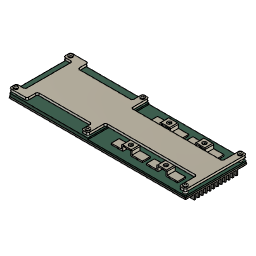
BMS (Autodesk Fusion 360 design; units mm, degrees)
Autodesk Fusion 360 part; units mm, degrees
note: some values were not read from the file. Set by a fixed rule: which sketch regions a step uses.
sketch "Sketch1" plane through (0, 0, 0) normal (0, 0, 1) x (1, 0, 0)
  line L0 (0, 0) -> (220, 0)
  line L1 (220, 0) -> (220, 76.5)
  line L2 (220, 76.5) -> (0, 76.5)
  line L3 (0, 76.5) -> (0, 0)
  line L4 (0, 38.25) -> (0, 65.25)
  line L5 (0, 38.25) -> (0, 11.25)
  line L6 (0, 11.25) -> (220, 11.25)
  line L7 (0, 65.25) -> (220, 65.25)
  line L8 (220, 0) -> (212, 0)
  line L9 (212, 0) -> (212, 76.5)
  line L10 (212, 38.25) -> (212, 54.25)
  line L11 (212, 38.25) -> (212, 22.25)
  line L12 (212, 22.25) -> (98, 22.25)
  line L13 (98, 22.25) -> (98, 54.25)
  line L14 (98, 54.25) -> (212, 54.25)
  line L15 (98, 54.25) -> (98, 76.5)
  line L16 (98, 22.25) -> (98, 0)
  line L17 (98, 0) -> (90, 0)
  line L18 (98, 76.5) -> (90, 76.5)
  line L19 (0, 0) -> (1.6578, 0)
  line L20 (0, 0) -> (22, 0)
  line L21 (0, 76.5) -> (22, 76.5)
  line L22 (22, 76.5) -> (22, 65.5)
  line L23 (24, 63.5) -> (88, 63.5)
  line L24 (90, 65.5) -> (90, 76.5)
  line L25 (22, 0) -> (22, 11)
  line L26 (24, 13) -> (88, 13)
  line L27 (90, 11) -> (90, 0)
  line L28 (0, 38.25) -> (0, 67.75)
  line L29 (0, 38.25) -> (0, 8.75)
  line L30 (0, 8.75) -> (9, 8.75)
  line L31 (11, 10.75) -> (11, 65.75)
  line L32 (9, 67.75) -> (0, 67.75)
  arc A0 (11, 65.75) -> (9, 67.75) centre (9, 65.75) ccw
  arc A1 (9, 8.75) -> (11, 10.75) centre (9, 10.75) ccw
  arc A2 (24, 13) -> (22, 11) centre (24, 11) ccw
  arc A3 (90, 11) -> (88, 13) centre (88, 11) ccw
  arc A4 (88, 63.5) -> (90, 65.5) centre (88, 65.5) ccw
  arc A5 (22, 65.5) -> (24, 63.5) centre (24, 65.5) ccw
  line L33 (94, 0) -> (94, 4)
  line L34 (0, 0) -> (4, 0)
  line L35 (4, 0) -> (4, 4)
  line L36 (4, 4) -> (0, 4)
  line L37 (0, 4) -> (0, 0)
  line L38 (216, 0) -> (216, 4)
  circle A6 centre (94, 4) radius 2.5
  circle A7 centre (4, 4) radius 2.5
  circle A8 centre (216, 4) radius 2.5
  line L39 (212, 76.5) -> (220, 76.5)
  line L40 (216, 76.5) -> (216, 72.5)
  circle A9 centre (216, 72.5) radius 2.5
  line L41 (94, 76.5) -> (94, 72.5)
  circle A10 centre (94, 72.5) radius 2.5
  line L42 (0, 76.5) -> (4, 76.5)
  line L43 (4, 76.5) -> (4, 72.5)
  line L44 (4, 72.5) -> (0, 72.5)
  line L45 (0, 72.5) -> (0, 76.5)
  circle A11 centre (4, 72.5) radius 2.5
  point P0 (22, 63.5)
  point P1 (22, 13)
  point P2 (11, 8.75)
  dimension "d1" = 220
  dimension "d2" = 76.5
  dimension "d3" = 27
  dimension "d4" = 27
  dimension "d5" = 8
  dimension "d6" = 16
  dimension "d7" = 16
  dimension "d8" = 114
  dimension "d9" = 8
  dimension "d10" = 8
  dimension "d11" = 22
  dimension "d12" = 22
  dimension "d13" = 13
  dimension "d14" = 13
  dimension "d15" = 29.5
  dimension "d16" = 29.5
  dimension "d17" = 11
  dimension "d18" = 2
  dimension "d19" = 4
  dimension "d20" = 4
  dimension "d21" = 4
  dimension "d22" = 4
  dimension "d23" = 5
  dimension "d24" = 5
  dimension "d25" = 5
  dimension "d26" = 4
  dimension "d27" = 5
  dimension "d28" = 4
  dimension "d29" = 5
  dimension "d30" = 4
  dimension "d31" = 4
  dimension "d32" = 5
  constraint horizontal L0
  constraint vertical L1
  constraint horizontal L2
  constraint vertical L3
  constraint coincident L0.start L3.end
  constraint midpoint L3 L4.start
  constraint parallel L3 L4
  constraint parallel L3 L5
  constraint coincident L1 L6.end
  constraint perpendicular L1 L6
  constraint coincident L1 L7.end
  constraint perpendicular L1 L7
  constraint perpendicular L1 L8
  constraint coincident L2 L9.end
  constraint perpendicular L2 L9
  constraint midpoint L9 L10.start
  constraint perpendicular L7 L10
  constraint parallel L9 L11
  constraint perpendicular L11 L12
  constraint perpendicular L6 L13
  constraint perpendicular L9 L14
  constraint coincident L2 L15.end
  constraint perpendicular L2 L15
  constraint coincident L0 L16.end
  constraint perpendicular L0 L16
  constraint coincident L0 L17.end
  constraint coincident L2 L18.end
  constraint coincident L0 L19.end
  constraint perpendicular L3 L20
  constraint perpendicular L3 L21
  constraint perpendicular L21 L22
  constraint perpendicular L22 L23
  constraint perpendicular L18 L24
  constraint perpendicular L6 L25
  constraint perpendicular L25 L26
  constraint perpendicular L17 L27
  constraint perpendicular L3 L30
  constraint perpendicular L7 L31
  constraint perpendicular L28 L32
  constraint tangent L31 A0
  constraint tangent L32 A0
  constraint coincident P2 L30
  constraint coincident P2 L31
  constraint tangent L30 A1
  constraint tangent L31 A1
  constraint equal A0 A1
  constraint coincident P1 L25
  constraint coincident P1 L26
  constraint tangent L25 A2
  constraint tangent L26 A2
  constraint equal A0 A2
  constraint tangent L26 A3
  constraint tangent L27 A3
  constraint equal A0 A3
  constraint tangent L23 A4
  constraint tangent L24 A4
  constraint equal A0 A4
  constraint coincident P0 L22
  constraint coincident P0 L23
  constraint tangent L22 A5
  constraint tangent L23 A5
  constraint equal A0 A5
  constraint midpoint L17 L33.start
  constraint perpendicular L0 L33
  constraint horizontal L34
  constraint vertical L35
  constraint horizontal L36
  constraint vertical L37
  constraint midpoint L8 L38.start
  constraint perpendicular L8 L38
  constraint coincident L33.end A6.centre
  constraint coincident L35.end L36.start
  constraint coincident L38.end A8.centre
  constraint midpoint L39 L40.start
  constraint perpendicular L39 L40
  constraint coincident L40.end A9.centre
  constraint midpoint L18 L41.start
  constraint perpendicular L18 L41
  constraint coincident L41.end A10.centre
  constraint horizontal L42
  constraint vertical L43
  constraint horizontal L44
  constraint vertical L45
  constraint coincident L43.end L44.start
  measures "d1" distance of L0.start L0.end
  measures "d2" distance of L0.start L2.end
  measures "d3" distance of L4.start L4.end
  measures "d4" distance of L4.start L5.end
  measures "d5" distance of L0.end L8.end
  measures "d6" distance of L10.start L10.end
  measures "d7" distance of L10.start L11.end
  measures "d8" distance of L11.end L12.end
  measures "d9" distance of L16.end L17.end
  measures "d10" distance of L15.end L18.end
  measures "d11" distance of L0.start L20.end
  measures "d12" distance of L2.end L21.end
  measures "d13" distance of L21.end P0
  measures "d14" distance of L20.end P1
  measures "d15" distance of L4.start L28.end
  measures "d16" distance of L4.start L29.end
  measures "d17" distance of L29.end P2
  measures "d18" radius of A0
  measures "d19" distance of L33.start L33.end
  measures "d20" distance of L0.start L34.end
  measures "d21" distance of L0.start L36.end
  measures "d22" distance of L38.start L38.end
  measures "d23" diameter of A6
  measures "d24" diameter of A7
  measures "d25" diameter of A8
  measures "d26" distance of L40.start L40.end
  measures "d27" diameter of A9
  measures "d28" distance of L41.start L41.end
  measures "d29" diameter of A10
  measures "d30" distance of L2.end L42.end
  measures "d31" distance of L2.end L44.end
  measures "d32" diameter of A11
extrude "Extrude1" add sketch "Sketch1" against normal blind 2 contours L0 L3 L19 L20 L34 L35 L36 L37 A7 | L0 L3 L6 L20 L25 L30 L31 A1 A2 L35 L36 A7 | L3 L6 L29 L30 L31 A1 | L35 L36 A7 | L35 L36 A7 | L0 L6 L25 L27 A2 A3 | L3 L4 L5 L6 L7 L28 L29 L31 | L0 L6 L16 L17 L27 A3 | L6 L7 L13 L15 L16 L23 L26 L31 A2 A3 A4 A5 | L6 L26 A2 A3 | L3 L7 L28 L31 L32 A0 | L2 L3 L7 L21 L22 L31 L32 A0 A5 L43 L44 A11 | L0 L6 L9 L16 | L2 L7 L22 L24 A4 A5 | L7 L23 A4 A5 | L0 L1 L6 L8 L9 | L6 L9 L12 L16 | L2 L3 L21 L42 L43 L44 L45 A11 | L2 L7 L15 L18 L24 A4 | L1 L6 L7 L9 L10 L11 | L9 L10 L11 L12 L13 L14 | L43 L44 A11 | L43 L44 A11 | L2 L7 L9 L15 | L7 L9 L14 L15 | L1 L2 L7 L9 L39 | A6 | A8 | A9 | A10 makes body 1
extrude "Extrude2" add sketch "Sketch1" along normal blind 4 and the other way blind -7 separate body contours L0 L3 L19 L20 L34 L35 L36 L37 A7 | L0 L3 L6 L20 L25 L30 L31 A1 A2 L35 L36 A7 | L35 L36 A7 | L35 L36 A7 | L0 L6 L16 L17 L27 A3 | L6 L7 L13 L15 L16 L23 L26 L31 A2 A3 A4 A5 | L2 L3 L7 L21 L22 L31 L32 A0 A5 L43 L44 A11 | L0 L1 L6 L8 L9 | L2 L3 L21 L42 L43 L44 L45 A11 | L2 L7 L15 L18 L24 A4 | L1 L6 L7 L9 L10 L11 | L9 L10 L11 L12 L13 L14 | L43 L44 A11 | L43 L44 A11 | L1 L2 L7 L9 L39 | A6 | A8 | A9 | A10 makes body 2
fillet "Fillet1" radius 2 18 edges at (98, 22.25, 5.5) (98, 54.25, 5.5) (212, 54.25, 5.5) (212, 22.25, 5.5) (212, 76.5, 5.5) (220, 76.5, 5.5) (212, 0, 5.5) (220, 0, 5.5) (98, 76.5, 5.5) (90, 76.5, 5.5) (98, 0, 5.5) (90, 0, 5.5) (22, 76.5, 5.5) (0, 76.5, 5.5) (0, 67.75, 5.5) (0, 8.75, 5.5) (0, 0, 5.5) (22, 0, 5.5) on bodies 2
extrude "Extrude3" add sketch "Sketch1" along normal blind 7 and the other way blind -9 contours L35 L36 A7 | L35 L36 A7 | L43 L44 A11 | L43 L44 A11 | A6 | A8 | A9 | A10 bodies 2
fillet "Fillet2" radius 1 6 edges at (1.6692, 71.596, 9) (1.6692, 3.096, 9) (91.6692, 3.096, 9) (91.6692, 71.596, 9) (213.6692, 3.096, 9) (213.6692, 71.596, 9) on bodies 2
extrude "Extrude4" add sketch "Sketch1" along normal blind 1.6 contours L0 L3 L19 L20 L34 L35 L36 L37 A7 | L0 L3 L6 L20 L25 L30 L31 A1 A2 L35 L36 A7 | L3 L6 L29 L30 L31 A1 | L35 L36 A7 | L35 L36 A7 | L0 L6 L25 L27 A2 A3 | L3 L4 L5 L6 L7 L28 L29 L31 | L0 L6 L16 L17 L27 A3 | L6 L7 L13 L15 L16 L23 L26 L31 A2 A3 A4 A5 | L6 L26 A2 A3 | L3 L7 L28 L31 L32 A0 | L2 L3 L7 L21 L22 L31 L32 A0 A5 L43 L44 A11 | L2 L7 L22 L24 A4 A5 | L7 L23 A4 A5 | L2 L3 L21 L42 L43 L44 L45 A11 | L2 L7 L15 L18 L24 A4 | L43 L44 A11 | L43 L44 A11 | A6 | A10 bodies 1
extrude "Extrude5" add sketch "Sketch1" along normal blind 4 contours L35 L36 A7 | L35 L36 A7 | L43 L44 A11 | L43 L44 A11 | A6 | A8 | A9 | A10 bodies 2
fillet "Fillet3" radius 1 4 edges at (220, 76.5, -1) (220, 0, -1) (0, 0, -1) (0, 76.5, -1) on bodies 1
extrude "Extrude6" add sketch "Sketch1" along normal blind -2 and the other way blind 4 separate body contours L0 L3 L19 L20 L34 L35 L36 L37 A7 | L0 L3 L6 L20 L25 L30 L31 A1 A2 L35 L36 A7 | L3 L6 L29 L30 L31 A1 | L35 L36 A7 | L35 L36 A7 | L0 L6 L25 L27 A2 A3 | L3 L4 L5 L6 L7 L28 L29 L31 | L0 L6 L16 L17 L27 A3 | L6 L7 L13 L15 L16 L23 L26 L31 A2 A3 A4 A5 | L6 L26 A2 A3 | L3 L7 L28 L31 L32 A0 | L2 L3 L7 L21 L22 L31 L32 A0 A5 L43 L44 A11 | L0 L6 L9 L16 | L2 L7 L22 L24 A4 A5 | L7 L23 A4 A5 | L0 L1 L6 L8 L9 | L6 L9 L12 L16 | L2 L3 L21 L42 L43 L44 L45 A11 | L2 L7 L15 L18 L24 A4 | L1 L6 L7 L9 L10 L11 | L9 L10 L11 L12 L13 L14 | L43 L44 A11 | L43 L44 A11 | L2 L7 L9 L15 | L7 L9 L14 L15 | L1 L2 L7 L9 L39 | A6 | A8 | A9 | A10 makes body 3
sketch "Sketch2" plane through (0, 0, -4) normal (0, 0, -1) x (1, 0, 0)
  line L0 (0, 0) -> (0, -76.5)
  line L1 (0, -76.5) -> (220, -76.5)
  line L2 (220, -76.5) -> (220, 0)
  line L3 (220, 0) -> (0, 0)
  line L4 (0, -38.25) -> (0, -11.25)
  line L5 (0, -38.25) -> (0, -65.25)
  line L6 (0, -65.25) -> (220, -65.25)
  line L7 (0, -11.25) -> (220, -11.25)
  line L8 (0, -65.25) -> (0, -63.5)
  line L9 (0, -63.5) -> (0, -60.5)
  line L10 (0, -60.5) -> (0, -58.75)
  line L11 (0, -58.75) -> (0, -55.75)
  line L12 (0, -55.75) -> (0, -54)
  line L13 (0, -54) -> (0, -51)
  line L14 (0, -51) -> (0, -49.25)
  line L15 (0, -49.25) -> (0, -46.25)
  line L16 (0, -46.25) -> (0, -44.5)
  line L17 (0, -44.5) -> (0, -41.5)
  line L18 (0, -41.5) -> (0, -39.75)
  line L19 (0, -39.75) -> (0, -38.25)
  line L20 (0, -11.25) -> (0, -13)
  line L21 (0, -13) -> (0, -16)
  line L22 (0, -16) -> (0, -17.75)
  line L23 (0, -17.75) -> (0, -20.75)
  line L24 (0, -20.75) -> (0, -22.5)
  line L25 (0, -22.5) -> (0, -25.5)
  line L26 (0, -25.5) -> (0, -27.25)
  line L27 (0, -27.25) -> (0, -30.25)
  line L28 (0, -30.25) -> (0, -32)
  line L29 (0, -32) -> (0, -35)
  line L30 (0, -35) -> (0, -36.75)
  line L31 (0, -63.5) -> (220, -63.5)
  line L32 (0, -60.5) -> (220, -60.5)
  line L33 (0, -58.75) -> (220, -58.75)
  line L34 (0, -55.75) -> (220, -55.75)
  line L35 (0, -54) -> (220, -54)
  line L36 (0, -51) -> (220, -51)
  line L37 (0, -49.25) -> (220, -49.25)
  line L38 (0, -46.25) -> (220, -46.25)
  line L39 (0, -44.5) -> (220, -44.5)
  line L40 (0, -41.5) -> (220, -41.5)
  line L41 (0, -39.75) -> (220, -39.75)
  line L42 (0, -13) -> (220, -13)
  line L43 (0, -16) -> (220, -16)
  line L44 (0, -17.75) -> (220, -17.75)
  line L45 (0, -20.75) -> (220, -20.75)
  line L46 (0, -22.5) -> (220, -22.5)
  line L47 (0, -25.5) -> (220, -25.5)
  line L48 (0, -27.25) -> (220, -27.25)
  line L49 (0, -30.25) -> (220, -30.25)
  line L50 (0, -32) -> (220, -32)
  line L51 (0, -35) -> (220, -35)
  line L52 (0, -36.75) -> (220, -36.75)
  dimension "d57" = 27
  dimension "d58" = 27
  dimension "d59" = 1.75
  dimension "d60" = 3
  dimension "d61" = 1.75
  dimension "d62" = 3
  dimension "d63" = 1.75
  dimension "d64" = 3
  dimension "d65" = 1.75
  dimension "d66" = 3
  dimension "d67" = 1.75
  dimension "d68" = 3
  dimension "d69" = 1.75
  dimension "d70" = 1.75
  dimension "d71" = 3
  dimension "d72" = 1.75
  dimension "d73" = 3
  dimension "d74" = 1.75
  dimension "d75" = 3
  dimension "d76" = 1.75
  dimension "d77" = 3
  dimension "d78" = 1.75
  dimension "d79" = 3
  dimension "d80" = 1.75
  constraint midpoint L0 L4.start
  constraint perpendicular L3 L4
  constraint perpendicular L3 L5
  constraint coincident L2 L6.end
  constraint perpendicular L2 L6
  constraint coincident L2 L7.end
  constraint perpendicular L2 L7
  constraint perpendicular L6 L8
  constraint parallel L5 L9
  constraint parallel L5 L10
  constraint parallel L5 L11
  constraint parallel L5 L12
  constraint parallel L5 L13
  constraint parallel L0 L14
  constraint parallel L5 L15
  constraint parallel L5 L16
  constraint parallel L5 L17
  constraint parallel L5 L18
  constraint perpendicular L7 L20
  constraint parallel L4 L21
  constraint parallel L4 L22
  constraint parallel L4 L23
  constraint coincident L0 L24.end
  constraint parallel L4 L25
  constraint parallel L4 L26
  constraint coincident L0 L27.end
  constraint parallel L4 L28
  constraint coincident L4 L29.end
  constraint coincident L4 L30.end
  constraint coincident L2 L31.end
  constraint perpendicular L2 L31
  constraint coincident L2 L32.end
  constraint perpendicular L2 L32
  constraint coincident L2 L33.end
  constraint perpendicular L2 L33
  constraint coincident L2 L34.end
  constraint perpendicular L2 L34
  constraint coincident L2 L35.end
  constraint perpendicular L2 L35
  constraint coincident L2 L36.end
  constraint perpendicular L2 L36
  constraint coincident L2 L37.end
  constraint perpendicular L2 L37
  constraint coincident L2 L38.end
  constraint perpendicular L2 L38
  constraint coincident L2 L39.end
  constraint perpendicular L2 L39
  constraint coincident L2 L40.end
  constraint perpendicular L2 L40
  constraint coincident L2 L41.end
  constraint perpendicular L2 L41
  constraint coincident L2 L42.end
  constraint perpendicular L2 L42
  constraint coincident L2 L43.end
  constraint perpendicular L2 L43
  constraint coincident L2 L44.end
  constraint perpendicular L2 L44
  constraint coincident L2 L45.end
  constraint perpendicular L2 L45
  constraint coincident L2 L46.end
  constraint perpendicular L2 L46
  constraint coincident L2 L47.end
  constraint perpendicular L2 L47
  constraint coincident L2 L48.end
  constraint perpendicular L2 L48
  constraint coincident L2 L49.end
  constraint perpendicular L2 L49
  constraint coincident L2 L50.end
  constraint perpendicular L2 L50
  constraint coincident L2 L51.end
  constraint perpendicular L2 L51
  constraint coincident L2 L52.end
  constraint perpendicular L2 L52
  measures "d57" distance of L4.start L4.end
  measures "d58" distance of L4.start L5.end
  measures "d59" distance of L5.end L8.end
  measures "d60" distance of L8.end L9.end
  measures "d61" distance of L9.end L10.end
  measures "d62" distance of L10.end L11.end
  measures "d63" distance of L11.end L12.end
  measures "d64" distance of L12.end L13.end
  measures "d65" distance of L13.end L14.end
  measures "d66" distance of L14.end L15.end
  measures "d67" distance of L15.end L16.end
  measures "d68" distance of L16.end L17.end
  measures "d69" distance of L17.end L18.end
  measures "d70" distance of L4.end L20.end
  measures "d71" distance of L20.end L21.end
  measures "d72" distance of L21.end L22.end
  measures "d73" distance of L22.end L23.end
  measures "d74" distance of L23.end L24.end
  measures "d75" distance of L24.end L25.end
  measures "d76" distance of L25.end L26.end
  measures "d77" distance of L26.end L27.end
  measures "d78" distance of L27.end L28.end
  measures "d79" distance of L28.end L29.end
  measures "d80" distance of L29.end L30.end
extrude "Extrude7" add sketch "Sketch2" along normal blind 6 and the other way blind 0 contours L0 L2 L4 L7 L20 L42 | L0 L2 L4 L22 L43 L44 | L0 L2 L4 L24 L45 L46 | L0 L2 L4 L26 L47 L48 | L0 L2 L4 L28 L49 L50 | L0 L2 L4 L30 L51 L52 | L0 L2 L5 L18 L40 L41 | L0 L2 L5 L16 L38 L39 | L0 L2 L5 L14 L36 L37 | L0 L2 L5 L12 L34 L35 | L0 L2 L5 L10 L32 L33 | L0 L2 L5 L6 L8 L31 bodies 3
sketch "Sketch3" plane through (0, 0, 7) normal (0, 0, 1) x (-1, 0, 0)
  circle A0 centre (-4, -72.5) radius 2.5
  circle A1 centre (-94, -4) radius 2.5
  circle A2 centre (-216, -4) radius 2.5
  circle A3 centre (-94, -72.5) radius 2.5
  circle A4 centre (-4, -4) radius 2.5
  circle A5 centre (-216, -72.5) radius 2.5
  arc A6 (-20, 0) -> (-22, -2) centre (-20, -2) ccw
  line L0 (-22, -2) -> (-22, -11)
  arc A7 (-24, -13) -> (-22, -11) centre (-24, -11) ccw
  line L1 (-24, -13) -> (-88, -13)
  arc A8 (-90, -11) -> (-88, -13) centre (-88, -11) ccw
  line L2 (-90, -11) -> (-90, -2)
  arc A9 (-90, -2) -> (-92, 0) centre (-92, -2) ccw
  line L3 (-92, 0) -> (-96, 0)
  arc A10 (-96, 0) -> (-98, -2) centre (-96, -2) ccw
  line L4 (-98, -2) -> (-98, -20.25)
  arc A11 (-100, -22.25) -> (-98, -20.25) centre (-100, -20.25) ccw
  line L5 (-100, -22.25) -> (-210, -22.25)
  arc A12 (-212, -20.25) -> (-210, -22.25) centre (-210, -20.25) ccw
  line L6 (-212, -20.25) -> (-212, -2)
  arc A13 (-212, -2) -> (-214, 0) centre (-214, -2) ccw
  line L7 (-214, 0) -> (-218, 0)
  arc A14 (-218, 0) -> (-220, -2) centre (-218, -2) ccw
  line L8 (-220, -2) -> (-220, -74.5)
  arc A15 (-220, -74.5) -> (-218, -76.5) centre (-218, -74.5) ccw
  line L9 (-218, -76.5) -> (-214, -76.5)
  arc A16 (-214, -76.5) -> (-212, -74.5) centre (-214, -74.5) ccw
  line L10 (-212, -74.5) -> (-212, -56.25)
  arc A17 (-210, -54.25) -> (-212, -56.25) centre (-210, -56.25) ccw
  line L11 (-210, -54.25) -> (-100, -54.25)
  arc A18 (-98, -56.25) -> (-100, -54.25) centre (-100, -56.25) ccw
  line L12 (-98, -56.25) -> (-98, -74.5)
  arc A19 (-98, -74.5) -> (-96, -76.5) centre (-96, -74.5) ccw
  line L13 (-96, -76.5) -> (-92, -76.5)
  arc A20 (-92, -76.5) -> (-90, -74.5) centre (-92, -74.5) ccw
  line L14 (-90, -74.5) -> (-90, -65.5)
  arc A21 (-88, -63.5) -> (-90, -65.5) centre (-88, -65.5) ccw
  line L15 (-88, -63.5) -> (-24, -63.5)
  arc A22 (-22, -65.5) -> (-24, -63.5) centre (-24, -65.5) ccw
  line L16 (-22, -65.5) -> (-22, -74.5)
  arc A23 (-22, -74.5) -> (-20, -76.5) centre (-20, -74.5) ccw
  line L17 (-20, -76.5) -> (-2, -76.5)
  arc A24 (-2, -76.5) -> (0, -74.5) centre (-2, -74.5) ccw
  line L18 (0, -74.5) -> (0, -69.75)
  arc A25 (0, -69.75) -> (-2, -67.75) centre (-2, -69.75) ccw
  line L19 (-2, -67.75) -> (-9, -67.75)
  arc A26 (-11, -65.75) -> (-9, -67.75) centre (-9, -65.75) ccw
  line L20 (-11, -65.75) -> (-11, -10.75)
  arc A27 (-9, -8.75) -> (-11, -10.75) centre (-9, -10.75) ccw
  line L21 (-9, -8.75) -> (-2, -8.75)
  arc A28 (-2, -8.75) -> (0, -6.75) centre (-2, -6.75) ccw
  line L22 (0, -6.75) -> (0, -2)
  arc A29 (0, -2) -> (-2, 0) centre (-2, -2) ccw
  line L23 (-2, 0) -> (-20, 0)
  line L24 (-98, -56.25) -> (-131, -56.25)
  line L25 (-212, -56.25) -> (-188, -56.25)
  line L26 (-188, -54.25) -> (-188, -57.25)
  line L27 (-131, -54.25) -> (-131, -57.25)
  line L28 (-188, -57.25) -> (-175, -57.25)
  line L29 (-131, -57.25) -> (-144, -57.25)
  line L30 (-188, -57.25) -> (-188, -67.25)
  line L31 (-188, -67.25) -> (-175, -67.25)
  line L32 (-175, -67.25) -> (-175, -57.25)
  line L33 (-131, -57.25) -> (-131, -67.25)
  line L34 (-131, -67.25) -> (-144, -67.25)
  line L35 (-144, -67.25) -> (-144, -57.25)
  line L36 (-220, -38.25) -> (-213, -38.25)
  line L37 (-188, -67.25) -> (-201, -67.25)
  line L38 (-201, -67.25) -> (-201, -57.25)
  line L39 (-201, -57.25) -> (-188, -57.25)
  line L40 (-175, -67.25) -> (-162, -67.25)
  line L41 (-162, -67.25) -> (-162, -57.25)
  line L42 (-162, -57.25) -> (-175, -57.25)
  line L43 (-144, -67.25) -> (-157, -67.25)
  line L44 (-157, -67.25) -> (-157, -57.25)
  line L45 (-157, -57.25) -> (-144, -57.25)
  line L46 (-131, -67.25) -> (-118, -67.25)
  line L47 (-118, -67.25) -> (-118, -57.25)
  line L48 (-118, -57.25) -> (-131, -57.25)
  line L49 (-157, -9.25) -> (-157, -19.25)
  line L50 (-144, -9.25) -> (-144, -19.25)
  line L51 (-188, -19.25) -> (-175, -19.25)
  line L52 (-131, -19.25) -> (-144, -19.25)
  line L53 (-175, -9.25) -> (-175, -19.25)
  line L54 (-157, -19.25) -> (-144, -19.25)
  line L55 (-131, -9.25) -> (-144, -9.25)
  line L56 (-201, -19.25) -> (-188, -19.25)
  line L57 (-131, -19.25) -> (-131, -9.25)
  line L58 (-118, -19.25) -> (-131, -19.25)
  line L59 (-118, -9.25) -> (-118, -19.25)
  line L60 (-131, -9.25) -> (-118, -9.25)
  line L61 (-201, -9.25) -> (-201, -19.25)
  line L62 (-162, -19.25) -> (-175, -19.25)
  line L63 (-162, -9.25) -> (-162, -19.25)
  line L64 (-188, -9.25) -> (-201, -9.25)
  line L65 (-175, -9.25) -> (-162, -9.25)
  line L66 (-188, -19.25) -> (-188, -9.25)
  line L67 (-144, -9.25) -> (-157, -9.25)
  line L68 (-188, -9.25) -> (-175, -9.25)
  line L69 (-188, -67.25) -> (-186.5, -67.25)
  line L70 (-186.5, -67.25) -> (-186.5, -57.25)
  line L71 (-175, -67.25) -> (-176.5, -67.25)
  line L72 (-176.5, -67.25) -> (-176.5, -57.25)
  line L73 (-144, -67.25) -> (-142.5, -67.25)
  line L74 (-142.5, -67.25) -> (-142.5, -57.25)
  line L75 (-131, -67.25) -> (-132.5, -67.25)
  line L76 (-132.5, -67.25) -> (-132.5, -57.25)
  line L77 (-188, -19.25) -> (-186.5, -19.25)
  line L78 (-186.5, -19.25) -> (-186.5, -9.25)
  line L79 (-175, -19.25) -> (-176.5, -19.25)
  line L80 (-176.5, -19.25) -> (-176.5, -9.25)
  line L81 (-144, -19.25) -> (-142.5, -19.25)
  line L82 (-142.5, -19.25) -> (-142.5, -9.25)
  line L83 (-131, -19.25) -> (-132.5, -19.25)
  line L84 (-132.5, -19.25) -> (-132.5, -9.25)
  circle A30 centre (-181.5, -62.25) radius 2.5
  circle A31 centre (-137.5, -62.25) radius 2.5
  circle A32 centre (-181.5, -14.25) radius 2.5
  circle A33 centre (-137.5, -14.25) radius 2.5
  dimension "d85" = 33
  dimension "d86" = 24
  dimension "d87" = 3
  dimension "d88" = 3
  dimension "d89" = 13
  dimension "d90" = 13
  dimension "d91" = 10
  dimension "d92" = 10
  dimension "d93" = 13
  dimension "d94" = 13
  dimension "d95" = 13
  dimension "d96" = 13
  dimension "d97" = 1.5
  dimension "d98" = 1.5
  dimension "d99" = 1.5
  dimension "d100" = 1.5
  dimension "d101" = 1.5
  dimension "d102" = 1.5
  dimension "d103" = 1.5
  dimension "d104" = 1.5
  dimension "d115" = 5
  dimension "d116" = 5
  dimension "d117" = 5
  dimension "d118" = 5
  constraint coincident A18.start L12.start
  constraint perpendicular L12 L24
  constraint coincident L10.end A17.end
  constraint perpendicular L10 L25
  constraint coincident L11 L26.start
  constraint perpendicular L11 L26
  constraint coincident L11 L27.start
  constraint perpendicular L24 L27
  constraint perpendicular L26 L28
  constraint perpendicular L27 L29
  constraint perpendicular L28 L30
  constraint perpendicular L26 L31
  constraint perpendicular L28 L32
  constraint perpendicular L29 L33
  constraint perpendicular L33 L34
  constraint perpendicular L29 L35
  constraint midpoint L8 L36.start
  constraint perpendicular L8 L36
  constraint perpendicular L30 L37
  constraint perpendicular L25 L38
  constraint perpendicular L38 L39
  constraint perpendicular L32 L40
  constraint perpendicular L28 L41
  constraint perpendicular L32 L42
  constraint perpendicular L35 L43
  constraint perpendicular L29 L44
  constraint perpendicular L44 L45
  constraint perpendicular L33 L46
  constraint perpendicular L29 L47
  constraint perpendicular L27 L48
  constraint symmetric L26.end L36 L51.start
  constraint symmetric L27.end L36 L52.start
  constraint symmetric L28.end L36 L51.end
  constraint symmetric L29.end L36 L50.end
  constraint symmetric L30.end L36 L64.start
  constraint symmetric L31.end L36 L53.start
  constraint symmetric L33.end L36 L55.start
  constraint symmetric L34.end L36 L50.start
  constraint symmetric L36 L37.end L61.start
  constraint symmetric L36 L38.end L56.start
  constraint symmetric L36 L40.end L63.start
  constraint symmetric L36 L41.end L62.start
  constraint symmetric L36 L43.end L49.start
  constraint symmetric L36 L44.end L49.end
  constraint symmetric L36 L46.end L59.start
  constraint symmetric L36 L47.end L58.start
  constraint perpendicular L30 L69
  constraint coincident L28 L70.end
  constraint perpendicular L28 L70
  constraint perpendicular L32 L71
  constraint coincident L28 L72.end
  constraint perpendicular L28 L72
  constraint perpendicular L35 L73
  constraint perpendicular L73 L74
  constraint perpendicular L33 L75
  constraint coincident L29 L76.end
  constraint perpendicular L29 L76
  constraint perpendicular L66 L77
  constraint coincident L68 L78.end
  constraint perpendicular L68 L78
  constraint perpendicular L53 L79
  constraint coincident L68 L80.end
  constraint perpendicular L68 L80
  constraint perpendicular L53 L81
  constraint coincident L55 L82.end
  constraint perpendicular L55 L82
  constraint perpendicular L57 L83
  constraint coincident L55 L84.end
  constraint perpendicular L55 L84
  measures "d85" distance of A18.start L24.end
  measures "d86" distance of L10.end L25.end
  measures "d87" distance of L26.start L26.end
  measures "d88" distance of L27.start L27.end
  measures "d89" distance of L26.end L28.end
  measures "d90" distance of L27.end L29.end
  measures "d91" distance of L26.end L30.end
  measures "d92" distance of L27.end L33.end
  measures "d93" distance of L30.end L37.end
  measures "d94" distance of L31.end L40.end
  measures "d95" distance of L34.end L43.end
  measures "d96" distance of L33.end L46.end
  measures "d97" distance of L30.end L69.end
  measures "d98" distance of L31.end L71.end
  measures "d99" distance of L34.end L73.end
  measures "d100" distance of L33.end L75.end
  measures "d101" distance of L51.start L77.end
  measures "d102" distance of L51.end L79.end
  measures "d103" distance of L50.end L81.end
  measures "d104" distance of L52.start L83.end
  measures "d115" diameter of A30
  measures "d116" diameter of A31
  measures "d117" diameter of A32
  measures "d118" diameter of A33
extrude "Extrude8" add sketch "Sketch3" along normal blind -7 and the other way blind 5.4 separate body contours L28 L30 L31 L69 L70 | L30 L37 L38 L39 | L28 L31 L32 L71 L72 | L32 L40 L41 L42 | L29 L33 L34 L75 L76 | L33 L46 L47 L48 | L29 L34 L35 L73 L74 | L35 L43 L44 L45 | L49 L50 L54 L67 | L50 L52 L55 L81 L82 | L52 L55 L57 L83 L84 | L57 L58 L59 L60 | L51 L66 L68 L77 L78 | L56 L61 L64 L66 | L51 L53 L68 L79 L80 | L53 L62 L63 L65 makes body 4 at (166.8333, 12.5833, 1.6) makes body 5 at (166.8333, 60.5833, 1.6) makes body 6 at (152.1667, 60.5833, 1.6) makes body 7 at (152.1667, 12.5833, 1.6) makes body 8 at (196.1667, 12.5833, 1.6) makes body 9 at (191.3333, 63.9167, 1.6) makes body 10 at (122.8333, 60.5833, 1.6) makes body 11 at (122.8333, 15.9167, 1.6)
extrude "Extrude9" add sketch "Sketch3" along normal blind -5.4 and the other way blind 0 contours L28 L30 L31 L69 L70 | L28 L31 L32 L71 L72 | L29 L33 L34 L75 L76 | L29 L34 L35 L73 L74 | L50 L52 L55 L81 L82 | L52 L55 L57 L83 L84 | L51 L66 L68 L77 L78 | L51 L53 L68 L79 L80 bodies 4 5 6 7 8 9 10 11
extrude "Extrude10" add sketch "Sketch3" against normal blind 1.5 contours L28 L31 L70 L72 | L29 L34 L74 L76 | L52 L55 L82 L84 | L51 L68 L78 L80 | A30 | A31 | A32 | A33 bodies 4 5 6 7 8 9 10 11
extrude "Extrude11" cut sketch "Sketch3" against normal blind 1.5 contours A30 | A31 | A32 | A33 bodies 4 5 6 7
fillet "Fillet4" radius 1 8 edges at (188, 14.25, 7) (175, 14.25, 7) (188, 62.25, 7) (175, 62.25, 7) (144, 62.25, 7) (131, 62.25, 7) (144, 14.25, 7) (131, 14.25, 7) on bodies 4 5 6 7
equation "d3 = ( 54 / 2 ) * 1 mm"
equation "d15 = ( 59 / 2 ) * 1 mm"
equation "d55 = -7.00 mm + 11 mm"
equation "d57 = ( 54 / 2 ) * 1 mm"
equation "d107 = 7.00 mm - 1.6 mm"
